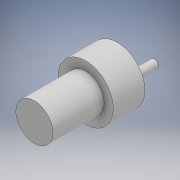
# Autodesk Inventor part: tamiya
Saved by Autodesk Inventor 2018 (Build 220112000, 112)
## iProperties
Created: 2019-04-04
Part Number: tamiya
Material: 一般
Document SubType Name: Modeling
Designer: Haruka
Density: 3.30451 g/cm^3
Appearance: 既定
Mass: 180 g
Surface Area: 97.406 cm^2
Volume: 54.471 cm^3
Author: Haruka
Autodesk Inventor part; units mm, degrees
ref_plane "YZ Plane" through (0, 0, 0) normal (1, 0, 0) x (0, 1, 0)
ref_plane "XZ Plane" through (0, 0, 0) normal (0, 1, 0) x (-1, 0, 0)
ref_plane "XY Plane" through (0, 0, 0) normal (0, 0, 1) x (1, 0, 0)
sketch "スケッチ1" plane through (0, 0, 0) normal (0, 1, 0) x (-1, 0, 0)
  circle A0 centre (0, 0) radius 20.5
  dimension "d0" = 41
  constraints: 1 centre point, 1 coincident
  measures "d0" diameter of A0
extrude "押し出し1" add sketch "スケッチ1" along normal blind 23.5
sketch "スケッチ2" plane through (0, 23.5, 0) normal (0, 1, 0) x (1, 0, 0)
  line L0 (0, 0) -> (7, 0)
  circle A0 centre (7, 0) radius 6
  dimension "d3" = 7
  dimension "d4" = 12
  constraints: 2 end point, 1 centre point, 1 coincident, 1 horizontal
  measures "d3" distance of L0.start L0.end
  measures "d4" diameter of A0
extrude "押し出し2" add sketch "スケッチ2" along normal blind 6
sketch "スケッチ3" plane through (7, 29.5, 0) normal (0, 1, 0) x (1, 0, 0)
  circle A0 centre (0, 0) radius 3
  point P0 (-7, 0)
  dimension "d7" = 6
  constraints: 1 centre point
  measures "d7" diameter of A0
extrude "押し出し3" add sketch "スケッチ3" along normal blind 15
sketch "スケッチ6" plane through (0, 23.5, 0) normal (0, 1, 0) x (1, 0, 0)
  circle A0 centre (0, 0) radius 15.5
  line L0 (0, 0) -> (23.5113, 0) construction
  line L1 (0, 0) -> (25.2681, -14.5885)
  line L2 (0, 0) -> (29.1771, 0) construction
  line L3 (0, 0) -> (-23.275, -13.4378)
  line L4 (0, 0) -> (26.8756, 0) construction
  point P0 (0, 15.5)
  point P1 (-13.4234, -7.75)
  point P2 (13.4234, -7.75)
  dimension "d31" = 31
  dimension "d33" = 30
  dimension "d34" = 150
  constraints: 10 end point, 3 horizontal, 3 point on circle, 2 equal length, 2 point on line, 1 centre point, 1 coincident
  measures "d31" diameter of A0
  measures "d33" angle of L1 L2
  measures "d34" angle of L3 L4
hole "穴3" at (0, 23.5, -15.5) at (-13.4234, 23.5, 7.75) at (13.4234, 23.5, 7.75) direction (0, -1, 0) diameter 3 depth 10 tip angle 118
sketch "スケッチ7" plane through (0, 0, 0) normal (0, -1, 0) x (1, 0, 0)
  circle A0 centre (0, 0) radius 13.75
  dimension "d42" = 27.5
  constraints: 1 centre point, 1 coincident
  measures "d42" diameter of A0
extrude "押し出し4" add sketch "スケッチ7" along normal blind 38
sketch "スケッチ8" plane through (7, 44.5, 0) normal (0, 1, 0) x (1, 0, 0)
  line L0 (-2.5, 0) -> (-2.5, 1.6583)
  circle A0 centre (0, 0) radius 3 projected
  line L1 (-2.5, 0) -> (-2.5, -1.6583)
  arc A1 (-2.5, 1.6583) -> (-2.5, -1.6583) centre (0, 0) ccw
  point P0 (-7, 0)
  constraints: 4 end point, 4 point on circle, 1 centre point, 1 concentric, 1 point on line
extrude "押し出し5" cut sketch "スケッチ8" against normal blind 7.5 contours L1 A0 L0 picked at (-2.6056, -0.897)
fillet "フィレット2" radius 0.5 1 edges at (7.866, 44.5, 2.8723)
